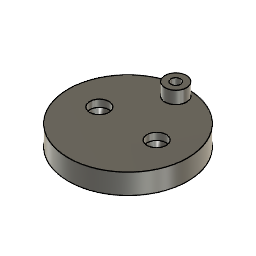
largage_moteur_bielle (Autodesk Fusion 360 design; units mm, degrees)
Autodesk Fusion 360 part; units mm, degrees
sketch "Esquisse1" plane through (0, 0, 0) normal (0, 0, 1) x (1, 0, 0)
  circle A0 centre (0, 0) radius 25
  circle A1 centre (-12, 0) radius 2.05
  circle A2 centre (12, 0) radius 2.05
  circle A3 centre (0, 20) radius 2
  dimension "d1" = 50
  dimension "d2" = 4.1
  dimension "d3" = 4.1
  dimension "d4" = 24
  dimension "d5" = 12
  dimension "d6" = 4
  dimension "d7" = 20
  constraint coincident A0.centre origin
  measures "d1" diameter of A0
  measures "d2" diameter of A1
  measures "d3" diameter of A2
  measures "d4" distance of A1.centre A2.centre
  measures "d5" distance of A0.centre A1.centre
  measures "d6" diameter of A3
  measures "d7" distance of A0.centre A3.centre
extrude "Extrusion1" add sketch "Esquisse1" along normal blind 8.5
sketch "Esquisse2" plane through (0, 0, 8.5) normal (0, 0, 1) x (-1, 0, 0)
  circle A0 centre (0, -20) radius 2
  circle A1 centre (-12, 0) radius 2.05
  circle A2 centre (12, 0) radius 2.05
  circle A3 centre (0, 0) radius 25
  circle A4 centre (0, -20) radius 4.5
  dimension "d10" = 9
  constraint concentric A0 A4
  measures "d10" diameter of A4
extrude "Extrusion2" add sketch "Esquisse2" along normal blind 5.2 contours A4
sketch "Esquisse3" plane through (0, 0, 8.5) normal (0, 0, 1) x (-1, 0, 0)
  circle A0 centre (0, -20) radius 4.5
  circle A1 centre (-12, 0) radius 2.05
  circle A2 centre (12, 0) radius 2.05
  circle A3 centre (0, 0) radius 25
  circle A4 centre (12, 0) radius 4
  circle A5 centre (-12, 0) radius 4
  dimension "d13" = 8
  dimension "d14" = 8
  constraint concentric A2 A4
  constraint concentric A1 A5
  measures "d13" diameter of A4
  measures "d14" diameter of A5
extrude "Extrusion3" cut sketch "Esquisse3" against normal blind 3 contours A4 | A5
hole "Perçage1" at (-12, 0, 5.5) direction (0, 0, -1) diameter 4 depth 10 tip angle 118 countersink diameter 8 countersink angle 90
hole "Perçage2" at (12, 0, 5.5) direction (0, 0, -1) diameter 4 depth 10 tip angle 118 countersink diameter 8 countersink angle 90
